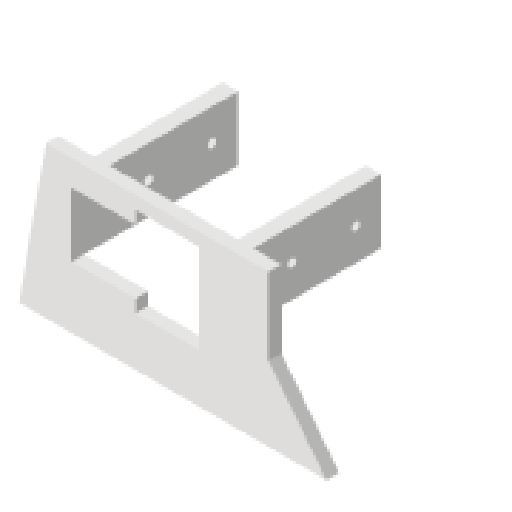
# Autodesk Inventor part: podstawa
Saved by Autodesk Inventor 2025.1 (Build 291241000, 241)
## iProperties
Created: 2025-03-27
Part Number: podstawa
Material: Ogólny
Document SubType Name: Modeling
Designer: Maciej
Density: 1 g/cm^3
Appearance: Domyślna
Author: Maciej
Autodesk Inventor part; units mm, degrees
ref_plane "YZ Plane" through (0, 0, 0) normal (1, 0, 0) x (0, 1, 0)
ref_plane "XZ Plane" through (0, 0, 0) normal (0, 1, 0) x (-1, 0, 0)
ref_plane "XY Plane" through (0, 0, 0) normal (0, 0, 1) x (1, 0, 0)
sketch "Szkic1" plane through (0, 0, 0) normal (0, 0, 1) x (1, 0, 0)
  line L0 (0, 0) -> (120, 0)
  line L1 (0, 0) -> (10.4189, 59.0885)
  line L2 (0, 0) -> (60, 0) construction
  line L3 (10.4189, 59.0885) -> (70.4189, 59.0885)
  line L4 (70.4189, 59.0885) -> (97.4189, 59.0885)
  line L5 (97.4189, 59.0885) -> (97.4189, 29.0885)
  line L6 (97.4189, 29.0885) -> (120, 0)
  line L7 (20.4189, 49.0885) -> (70.4189, 49.0885)
  line L8 (70.4189, 49.0885) -> (70.4189, 24.0885)
  line L9 (70.4189, 24.0885) -> (20.4189, 24.0885)
  line L10 (20.4189, 24.0885) -> (20.4189, 49.0885)
  dimension "d0" = 120
  dimension "d1" = 60
  dimension "d2" = 80
  dimension "d3" = 60
  dimension "d4" = 27
  dimension "d5" = 30
  dimension "d6" = 50
  dimension "d7" = 25
  dimension "d8" = 10
  dimension "d9" = 10
  constraints: 22 end point, 5 horizontal, 2 parallel, 2 perpendicular, 1 equal length
  measures "d0" distance of L0.start L0.end
  measures "d1" distance of L0.start L1.end
  measures "d2" angle of L2 L1
  measures "d3" distance of L1.end L3.end
  measures "d4" distance of L3.end L4.end
  measures "d5" distance of L4.end L5.end
  measures "d6" distance of L8.end L9.end
  measures "d7" distance of L7.end L8.end
  measures "d8" distance from line of L3 L7.start
  measures "d9" horizontal distance of L1.end L7.start
extrude "Wyciągnięcie proste1" add sketch "Szkic1" along normal blind 5
sketch "Szkic2" plane through (0, 0, 0) normal (0, 0, -1) x (-1, 0, 0)
  line L0 (-20.4189, 24.0885) -> (-20.4189, 49.0885) projected
  line L1 (-20.4189, 49.0885) -> (-14.4189, 49.0885)
  line L2 (-14.4189, 49.0885) -> (-14.4189, 24.0885)
  line L3 (-14.4189, 24.0885) -> (-20.4189, 24.0885)
  line L4 (-20.4189, 24.0885) -> (-20.4189, 49.0885)
  point P0 (0, 0)
  dimension "d12" = 6
  constraints: 8 end point, 2 parallel, 1 horizontal, 1 perpendicular
  measures "d12" distance of L2.end L3.end
extrude "Wyciągnięcie proste2" add sketch "Szkic2" along normal blind 30
sketch "Szkic3" plane through (0, 0, -30) normal (0, 0, -1) x (-1, 0, 0)
  line L0 (-20.4189, 24.0885) -> (-20.4189, 49.0885) projected
  line L1 (-20.4189, 24.0885) -> (-14.4189, 24.0885) projected
  line L2 (-20.4189, 49.0885) -> (-14.4189, 49.0885)
  line L3 (-14.4189, 49.0885) -> (-14.4189, 24.0885)
  line L4 (-14.4189, 24.0885) -> (-20.4189, 24.0885)
  line L5 (-20.4189, 24.0885) -> (-20.4189, 49.0885)
  point P0 (0, 0)
  constraints: 8 end point, 2 parallel, 1 horizontal, 1 perpendicular
extrude "Wyciągnięcie proste3" add sketch "Szkic3" along normal blind 30
sketch "Szkic4" plane through (0, 0, 0) normal (0, 0, -1) x (-1, 0, 0)
  line L0 (-70.4189, 49.0885) -> (-70.4189, 24.0885) projected
  line L1 (-70.4189, 49.0885) -> (-76.4189, 49.0885)
  line L2 (-76.4189, 49.0885) -> (-76.4189, 24.0885)
  line L3 (-76.4189, 24.0885) -> (-70.4189, 24.0885)
  line L4 (-70.4189, 24.0885) -> (-70.4189, 49.0885)
  point P0 (0, 0)
  dimension "d17" = 6
  constraints: 8 end point, 2 parallel, 1 horizontal, 1 perpendicular
  measures "d17" distance of L3.end L2.end
extrude "Wyciągnięcie proste4" add sketch "Szkic4" along normal up to surface (60 mm away)
sketch "Szkic5" plane through (14.4189, 24.0885, 0) normal (-1, 0, 0) x (0, 0, 1)
  line L0 (-60, 0) -> (-60, 25) projected
  point P0 (0, -24.0885)
  point P1 (-50, 12.5)
  point P2 (-60, 12.5)
  dimension "d20" = 10
  constraints: 1 midpoint
  measures "d20" distance of point (-60, 12.5) point (-50, 12.5)
hole "Otwór1" at (14.4189, 36.5885, -50) direction (1, 0, 0) diameter 3.5 depth 6
sketch "Szkic7" plane through (76.4189, 24.0885, 0) normal (1, 0, 0) x (0, 0, -1)
  circle A0 centre (50, 12.5) radius 1.75 projected
  point P0 (0, -24.0885)
  constraints: 1 coincident
hole "Otwór2" at (76.4189, 36.5885, -50) direction (-1, 0, 0) diameter 3.5 depth 6
sketch "Szkic8" plane through (14.4189, 24.0885, 0) normal (-1, 0, 0) x (0, 0, 1)
  point P0 (0, -24.0885)
  point P1 (-25.1365, 12.5)
hole "Otwór3" at (14.4189, 36.5885, -25.1365) direction (1, 0, 0) diameter 3.4 end through all clearance for "Śruba ze łbem stożkowym ISO 2009/7046" size "M3" standard "ISO"
sketch "Szkic10" plane through (0, 0, 0) normal (0, 0, -1) x (-1, 0, 0)
  line L0 (-70.4189, 49.0885) -> (-70.4189, 24.0885) projected
  line L1 (-70.4189, 49.0885) -> (-70.4189, 54.0885)
  line L2 (-70.4189, 54.0885) -> (-45.4189, 54.0885)
  line L3 (-70.4189, 24.0885) -> (-70.4189, 19.0885)
  line L4 (-70.4189, 19.0885) -> (-45.4189, 19.0885)
  line L5 (-45.4189, 19.0885) -> (-45.4189, 54.0885)
  point P0 (0, 0)
  dimension "d49" = 5
  dimension "d50" = 5
  constraints: 10 end point, 2 perpendicular, 2 vertical, 1 horizontal
  measures "d49" distance of L0.start L1.end
  measures "d50" distance of L0.end L3.end
extrude "Wyciągnięcie proste7" cut sketch "Szkic10" against normal blind 10
